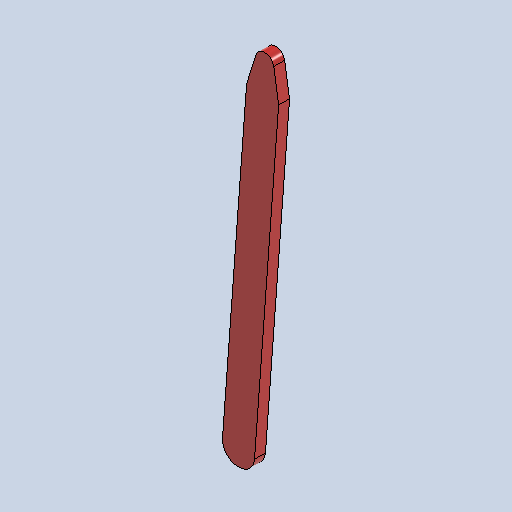
# Autodesk Inventor part: Triple Indexer band
Saved by Autodesk Inventor 2023.2 (Build 272271030, 271C)
## iProperties
Created: 2023-04-07
Part Number: Triple Indexer band
Material: Generic
Document SubType Name: Modeling
Designer: Main Account
Density: 1 g/cm^3
Appearance: Default
Author: Main Account
Autodesk Inventor part; units mm, degrees
ref_plane "YZ Plane" through (0, 0, 0) normal (1, 0, 0) x (0, 1, 0)
ref_plane "XZ Plane" through (0, 0, 0) normal (0, 1, 0) x (-1, 0, 0)
ref_plane "XY Plane" through (0, 0, 0) normal (0, 0, 1) x (1, 0, 0)
sketch "Sketch1" plane through (0, 0, 0) normal (0, 0, 1) x (1, 0, 0)
  circle A0 centre (6, 6) radius 6.35 construction
  arc A1 (-0.3319, 6.4786) -> (12.3319, 5.5214) centre (6, 6) ccw
  circle A2 centre (18.014, 164.9586) radius 6.35 construction
  arc A3 (21.1505, 165.4512) -> (14.9871, 165.917) centre (18.014, 164.9586) ccw
  line L0 (10.6933, 152.3554) -> (10.6053, 151.1903) construction
  line L1 (23.3572, 151.3983) -> (23.2691, 150.2332) construction
  line L2 (23.3572, 151.3983) -> (21.1505, 165.4512)
  line L3 (14.9871, 165.917) -> (10.6933, 152.3554)
  line L4 (23.3572, 151.3983) -> (23.2691, 150.2332)
  line L5 (10.6933, 152.3554) -> (10.6053, 151.1903)
  line L6 (10.6053, 151.1903) -> (-0.3319, 6.4786)
  line L7 (12.3319, 5.5214) -> (23.2691, 150.2332)
  line L8 (13.35, 129.2896) -> (13.35, 130.5741)
  line L9 (-1.35, 130.5741) -> (-1.35, 129.2896)
  line L10 (24.2663, 150.1578) -> (24.3631, 151.4387)
  line L11 (24.3631, 151.4387) -> (22.1384, 165.6063)
  arc A4 (22.1384, 165.6063) -> (14.0337, 166.2188) centre (18.014, 164.9586) ccw
  line L12 (14.0337, 166.2188) -> (9.7049, 152.5466)
  line L13 (9.7049, 152.5466) -> (9.6081, 151.2657)
  line L14 (9.6081, 151.2657) -> (-1.3291, 6.5539)
  arc A5 (-1.3291, 6.5539) -> (13.3291, 5.4461) centre (6, 6) ccw
  line L15 (13.3291, 5.4461) -> (24.2663, 150.1578)
  point P0 (0, 0)
  point P1 (8.8484, 141.2146)
  point P2 (9.2772, 146.8874)
  point P3 (8.2267, 132.9885)
  point P4 (9.9854, 148.4188)
  point P5 (10.4028, 148.5118)
  point P6 (9.4615, 149.3265)
  point P7 (8.8484, 141.2146)
  point P8 (9.2772, 146.8874)
  dimension "d0" = 6.35
  dimension "d5" = 1
  constraints: 28 end point, 8 point on circle, 4 centre point, 4 tangent, 2 coincident, 2 collinear, 1 concentric, 7 other
  measures "d0" diameter of A3
  measures "d5" distance between parallel lines of L7 L15
extrude "Extrusion1" add sketch "Sketch1" along normal blind 5 contours L6 L5 L3 A3 L2 L4 L7 A1 | L15 A5 L14 L13 L12 A4 L11 L10
body "Solid1"
